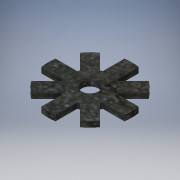
# Autodesk Inventor part: Tooth Disc
Saved by Autodesk Inventor 2019 (Build 230136000, 136)
## iProperties
Created: 2020-01-31
Part Number: Tooth Disc
Material: Steel
Document SubType Name: Modeling
Designer: alb16148
Density: 7.85 g/cm^3
Appearance: Plate
Author: alb16148
Autodesk Inventor part; units mm, degrees
ref_plane "YZ Plane" through (0, 0, 0) normal (1, 0, 0) x (0, 1, 0)
ref_plane "XZ Plane" through (0, 0, 0) normal (0, 1, 0) x (-1, 0, 0)
ref_plane "XY Plane" through (0, 0, 0) normal (0, 0, 1) x (1, 0, 0)
sketch "Sketch1" plane through (0, 0, 0) normal (0, 1, 0) x (-1, 0, 0)
  circle A0 centre (0, 0) radius 3
  circle A1 centre (0, 0) radius 15 construction
  line L0 (14.7902, 2.5) -> (7.0711, 2.5)
  line L1 (14.7902, -2.5) -> (7.0711, -2.5)
  arc A2 (14.7902, -2.5) -> (14.7902, 2.5) centre (0, 0) ccw
  line L2 (8.6905, 12.226) -> (3.2322, 6.7678)
  arc A3 (12.226, 8.6905) -> (8.6905, 12.226) centre (0, 0) ccw
  line L3 (12.226, 8.6905) -> (6.7678, 3.2322)
  line L4 (-2.5, 14.7902) -> (-2.5, 7.0711)
  arc A4 (2.5, 14.7902) -> (-2.5, 14.7902) centre (0, 0) ccw
  line L5 (2.5, 14.7902) -> (2.5, 7.0711)
  line L6 (-12.226, 8.6905) -> (-6.7678, 3.2322)
  arc A5 (-8.6905, 12.226) -> (-12.226, 8.6905) centre (0, 0) ccw
  line L7 (-8.6905, 12.226) -> (-3.2322, 6.7678)
  line L8 (-14.7902, -2.5) -> (-7.0711, -2.5)
  arc A6 (-14.7902, 2.5) -> (-14.7902, -2.5) centre (0, 0) ccw
  line L9 (-14.7902, 2.5) -> (-7.0711, 2.5)
  line L10 (-8.6905, -12.226) -> (-3.2322, -6.7678)
  arc A7 (-12.226, -8.6905) -> (-8.6905, -12.226) centre (0, 0) ccw
  line L11 (-12.226, -8.6905) -> (-6.7678, -3.2322)
  line L12 (2.5, -14.7902) -> (2.5, -7.0711)
  arc A8 (-2.5, -14.7902) -> (2.5, -14.7902) centre (0, 0) ccw
  line L13 (-2.5, -14.7902) -> (-2.5, -7.0711)
  line L14 (12.226, -8.6905) -> (6.7678, -3.2322)
  arc A9 (8.6905, -12.226) -> (12.226, -8.6905) centre (0, 0) ccw
  line L15 (8.6905, -12.226) -> (3.2322, -6.7678)
  arc A10 (6.7678, -3.2322) -> (7.0711, -2.5) centre (0, 0) ccw
  arc A11 (2.5, -7.0711) -> (3.2322, -6.7678) centre (0, 0) ccw
  arc A12 (-3.2322, -6.7678) -> (-2.5, -7.0711) centre (0, 0) ccw
  arc A13 (-7.0711, -2.5) -> (-6.7678, -3.2322) centre (0, 0) ccw
  arc A14 (-6.7678, 3.2322) -> (-7.0711, 2.5) centre (0, 0) ccw
  arc A15 (-2.5, 7.0711) -> (-3.2322, 6.7678) centre (0, 0) ccw
  arc A16 (7.0711, 2.5) -> (6.7678, 3.2322) centre (0, 0) ccw
  arc A17 (3.2322, 6.7678) -> (2.5, 7.0711) centre (0, 0) ccw
  circle A18 centre (0, 0) radius 7.5 construction
  dimension "d8" = 15
  dimension "d0" = 6
  dimension "d1" = 30
  dimension "d3" = 5
  dimension "d6" = 360
  constraints: 34 point on circle, 32 end point, 18 centre point, 5 coincident, 2 horizontal, 1 vertical alignment, 68 other
  measures "d0" diameter of A0
  measures "d1" diameter of A1
  measures "d3" distance between parallel lines of L1 L0
extrude "Extrusion1" add sketch "Sketch1" along normal blind 2
body "Solid1"
